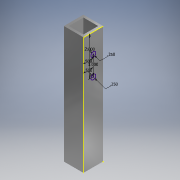
# Autodesk Inventor part: 15102898-16-P-0912
Saved by Autodesk Inventor 2017 (Build 210142000, 142)
## iProperties
Created: 2016-10-13
Part Number: 15102898-16-P-0912
Material: Aluminum 6061
Document SubType Name: Modeling
Designer: 15102898
Density: 2.7 g/cm^3
Appearance: Aluminum - Flat
Author: 15102898
Autodesk Inventor part; units mm, degrees
ref_plane "YZ Plane" through (0, 0, 0) normal (1, 0, 0) x (0, 1, 0)
ref_plane "XZ Plane" through (0, 0, 0) normal (0, 1, 0) x (-1, 0, 0)
ref_plane "XY Plane" through (0, 0, 0) normal (0, 0, 1) x (1, 0, 0)
sketch "Sketch1" plane through (0, 0, 0) normal (0, 1, 0) x (-1, 0, 0)
  line L0 (0, 0) -> (25.4, 0)
  line L1 (25.4, 0) -> (25.4, 25.4)
  line L2 (25.4, 25.4) -> (0, 25.4)
  line L3 (0, 25.4) -> (0, 0)
  line L4 (22.225, 22.225) -> (3.175, 22.225)
  line L5 (3.175, 22.225) -> (3.175, 3.175)
  line L6 (3.175, 3.175) -> (22.225, 3.175)
  line L7 (22.225, 3.175) -> (22.225, 22.225)
  dimension "d0" = 25.4
  dimension "d1" = 25.4
  dimension "d2" = 3.175
  dimension "d3" = 3.175
  dimension "d4" = 3.175
  dimension "d5" = 3.175
  constraints: 16 end point, 4 parallel, 2 horizontal, 2 perpendicular
  measures "d0" distance of L2.end L1.end
  measures "d1" distance of L1.end L0.end
  measures "d2" distance between parallel lines of L1 L7
  measures "d3" distance between parallel lines of L0 L6
  measures "d4" distance between parallel lines of L2 L4
  measures "d5" distance between parallel lines of L3 L5
extrude "Extrusion1" add sketch "Sketch1" along normal blind 152.4
sketch "Sketch2" plane through (0, 0, 25.4) normal (1, 0, 0) x (0, 0, -1)
  circle A0 centre (12.7, 114.3) radius 3.175
  circle A1 centre (12.7, 88.9) radius 3.175
  line L0 (0, 0) -> (0, 152.4) projected
  line L1 (0, 152.4) -> (25.4, 152.4) projected
  point P0 (25.4, 0)
  dimension "d8" = 12.7
  dimension "d10" = 12.7
  dimension "d11" = 25.4
  dimension "d12" = 6.35
  dimension "d13" = 6.35
  dimension "d14" = 38.1
  constraints: 2 centre point
  measures "d8" distance from line of L0 A1.centre
  measures "d10" distance from line of L0 A0.centre
  measures "d11" distance of A1.centre A0.centre
  measures "d12" diameter of A0
  measures "d13" diameter of A1
  measures "d14" distance from line of L1 A0.centre
extrude "Extrusion2" cut sketch "Sketch2" against normal blind 25.4
sketch "Sketch3" plane through (-25.4, 0, 25.4) normal (0, 0, 1) x (1, 0, 0)
  circle A0 centre (12.7, 12.7) radius 3.175
  line L0 (0, 0) -> (0, 152.4) projected
  line L1 (0, 0) -> (25.4, 0) projected
  dimension "d17" = 6.35
  dimension "d18" = 12.7
  dimension "d19" = 12.7
  constraints: 1 centre point
  measures "d17" diameter of A0
  measures "d18" distance from line of L0 A0.centre
  measures "d19" distance from line of L1 A0.centre
extrude "Extrusion3" cut sketch "Sketch3" against normal blind 25.4
body "Solid1"
